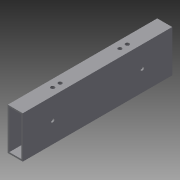
# Autodesk Inventor part: 000101
Saved by Autodesk Inventor 2015 (Build 190159000, 159)
## iProperties
Created: 2015-05-11
Part Number: 000101
Material: Generic
Document SubType Name: Modeling
Designer: Wesley
Density: 1 g/cm^3
Appearance: Default
Author: Wesley
Autodesk Inventor part; units mm, degrees
ref_plane "YZ Plane" through (0, 0, 0) normal (1, 0, 0) x (0, 1, 0)
ref_plane "XZ Plane" through (0, 0, 0) normal (0, 1, 0) x (-1, 0, 0)
ref_plane "XY Plane" through (0, 0, 0) normal (0, 0, 1) x (1, 0, 0)
sketch "Sketch1" plane through (0, 0, 0) normal (0, 0, 1) x (1, 0, 0)
  line L0 (0, 0) -> (12.7, 0)
  line L1 (12.7, 0) -> (12.7, 35.56)
  line L2 (12.7, 35.56) -> (0, 35.56)
  line L3 (0, 35.56) -> (0, 0)
  line L4 (1.27, 34.29) -> (11.43, 34.29)
  line L5 (11.43, 34.29) -> (11.43, 1.27)
  line L6 (11.43, 1.27) -> (1.27, 1.27)
  line L7 (1.27, 1.27) -> (1.27, 34.29)
  dimension "d0" = 35.56
  dimension "d1" = 12.7
  dimension "d2" = 1.27
  constraints: 16 end point, 4 parallel, 2 perpendicular, 1 horizontal, 3 other
  measures "d0" distance of L2.end L0.start
  measures "d1" distance of L0.start L0.end
  measures "d2" distance between parallel lines of L2 L4
extrude "Extrusion1" add sketch "Sketch1" along normal blind 127
sketch "Sketch2" plane through (12.7, 0, 0) normal (1, 0, 0) x (0, 0, -1)
  line L0 (-168.1044, 17.78) -> (-15.152, 17.78) construction
  line L1 (0, 0) -> (-127, 0) construction
  line L2 (-127, 0) -> (-127, 35.56) projected
  line L3 (0, 0) -> (0, 35.56) projected
  point P0 (-101.6, 17.78)
  point P1 (-25.4, 17.78)
  dimension "d5" = 17.78
  dimension "d6" = 25.4
  dimension "d7" = 25.4
  constraints: 2 end point, 2 point on line, 1 horizontal
  measures "d5" distance between parallel lines of L1 L0
  measures "d6" distance from line of L2 point (-101.6, 17.78)
  measures "d7" distance from line of L3 point (-25.4, 17.78)
hole "Hole1" at (12.7, 17.78, 101.6) at (12.7, 17.78, 25.4) direction (-1, 0, 0) diameter 3.2639 end through all
sketch "Sketch4" plane through (0, 35.56, 0) normal (0, 1, 0) x (1, 0, 0)
  line L0 (6.35, 23.2485) -> (6.35, -226.9955) construction
  line L1 (12.7, 0) -> (12.7, -127) construction
  line L2 (12.7, 0) -> (0, 0) projected
  line L3 (0, 0) -> (0, -127) projected
  line L4 (12.7, -127) -> (0, -127) projected
  line L5 (12.7, 0) -> (12.7, -127) projected
  point P0 (0, 0)
  point P1 (6.35, -31.75)
  point P2 (6.35, -95.25)
  dimension "d27" = 6.35
  dimension "d28" = 31.75
  dimension "d29" = 31.75
  constraints: 2 end point, 2 point on line, 1 vertical
  measures "d27" distance between parallel lines of L1 L0
  measures "d28" distance from line of L2 point (6.35, -31.75)
  measures "d29" distance from line of L4 point (6.35, -95.25)
hole "Hole3" at (6.35, 35.56, 31.75) at (6.35, 35.56, 95.25) direction (0, -1, 0) diameter 3.2512 end through all
sketch "Sketch5" plane through (0, 35.56, 0) normal (0, 1, 0) x (1, 0, 0)
  line L0 (-68.5901, -63.5) -> (110.3325, -63.5) construction
  line L1 (12.7, -127) -> (0, -127) construction
  line L2 (-35.2645, -38.1) -> (103.538, -38.1) construction
  line L3 (-49.1771, -88.9) -> (128.7748, -88.9) construction
  line L4 (6.35, 12.1996) -> (6.35, -141.0127) construction
  line L5 (0, 0) -> (0, -127) construction
  point P0 (6.35, -38.1)
  point P1 (6.35, -88.9)
  dimension "d37" = 63.5
  dimension "d38" = 25.4
  dimension "d39" = 25.4
  dimension "d40" = 6.35
  constraints: 8 end point, 4 point on line, 3 horizontal, 1 vertical
  measures "d37" distance between parallel lines of L1 L0
  measures "d38" distance between parallel lines of L0 L2
  measures "d39" distance between parallel lines of L3 L0
  measures "d40" distance between parallel lines of L5 L4
hole "Hole4" at (6.35, 35.56, 38.1) at (6.35, 35.56, 88.9) direction (0, -1, 0) diameter 3.175 end through all
body "Solid1"
